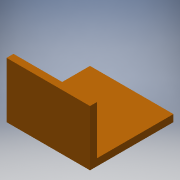
# Autodesk Inventor part: angle bracket
Saved by Autodesk Inventor 2017 SP1 (Build 210196100, 196)
## iProperties
Created: 2018-01-24
Part Number: angle bracket
Material: Aluminum 6061
Document SubType Name: Modeling
Designer: Ben
Density: 2.7 g/cm^3
Appearance: Orange
Author: Ben
Autodesk Inventor part; units mm, degrees
ref_plane "YZ Plane" through (0, 0, 0) normal (1, 0, 0) x (0, 1, 0)
ref_plane "XZ Plane" through (0, 0, 0) normal (0, 1, 0) x (-1, 0, 0)
ref_plane "XY Plane" through (0, 0, 0) normal (0, 0, 1) x (1, 0, 0)
sketch "Sketch1" plane through (0, 0, 0) normal (1, 0, 0) x (0, 1, 0)
  line L0 (0, 0) -> (25.4, 0)
  line L1 (25.4, 0) -> (25.4, -3.175)
  line L2 (25.4, -3.175) -> (3.175, -3.175)
  line L3 (3.175, -3.175) -> (3.175, -38.1)
  line L4 (3.175, -38.1) -> (0, -38.1)
  line L5 (0, -38.1) -> (0, 0)
  dimension "d0" = 25.4
  dimension "d1" = 3.175
  dimension "d4" = 38.1
  constraints: 12 end point, 6 perpendicular, 1 horizontal
  measures "d0" distance of L0.start L0.end
  measures "d1" distance of L3.end L4.end
  measures "d4" distance of L4.end L0.start
extrude "Extrusion1" add sketch "Sketch1" along normal blind 38.1
sketch "Sketch2" plane through (0, 0, -38.1) normal (0, -1, 0) x (1, 0, 0)
  circle A0 centre (19.05, 15.875) radius 4.7625
  line L0 (38.1, 38.1) -> (38.1, 0) projected
  point P0 (0, 38.1)
  dimension "d5" = 9.525
  dimension "d6" = 22.225
  dimension "d7" = 19.05
  constraints: 1 centre point
  measures "d5" diameter of A0
  measures "d6" vertical distance of point (0, 38.1) A0.centre
  measures "d7" distance from line of A0.centre L0
extrude "Extrusion2" cut sketch "Sketch2" against normal through all
body "Solid1"
